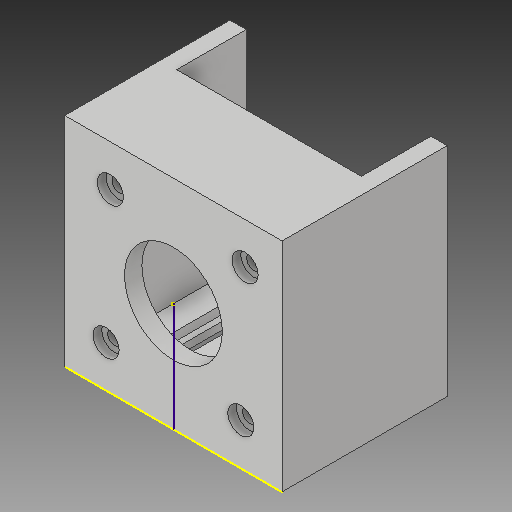
# Autodesk Inventor part: stepperMount
Saved by Autodesk Inventor 2017 (Build 210142000, 142)
## iProperties
Created: 2017-04-11
Part Number: stepperMount
Material: Generic
Document SubType Name: Modeling
Designer: Andres Celi
Density: 1 g/cm^3
Appearance: Default
Author: Andres Celi
Autodesk Inventor part; units mm, degrees
ref_plane "YZ Plane" through (0, 0, 0) normal (1, 0, 0) x (0, 1, 0)
ref_plane "XZ Plane" through (0, 0, 0) normal (0, 1, 0) x (-1, 0, 0)
ref_plane "XY Plane" through (0, 0, 0) normal (0, 0, 1) x (1, 0, 0)
sketch "Sketch1" plane through (0, 0, 0) normal (0, 0, 1) x (1, 0, 0)
  point P0 (0, 0)
sketch "Sketch2" plane through (0, 0, 0) normal (0, 0, 1) x (1, 0, 0)
  line L0 (-25, 25) -> (25, 25)
  line L1 (25, 25) -> (25, -25)
  line L2 (25, -25) -> (-25, -25)
  line L3 (-25, -25) -> (-25, 25)
  point P0 (0, 0)
  dimension "d0" = 50
  dimension "d1" = 50
  dimension "d2" = 25
  dimension "d3" = 25
  constraints: 8 end point, 2 parallel, 1 horizontal, 1 perpendicular
  measures "d0" distance of L1.end L2.end
  measures "d1" distance of L0.end L1.end
  measures "d2" distance from line of L3 point (0, 0)
  measures "d3" distance from line of point (0, 0) L0
extrude "Extrusion1" add sketch "Sketch2" along normal blind 38
sketch "Sketch3" plane through (0, 0, 0) normal (0, 0, -1) x (-1, 0, 0)
  point P0 (0, 0)
sketch "Sketch4" plane through (-25, 25, 0) normal (0, 1, 0) x (1, 0, 0)
  line L0 (0, 0) -> (50, 0) projected
  line L1 (46.25, 0) -> (3.75, 0)
  line L2 (3.75, 0) -> (3.75, -16)
  line L3 (3.75, -16) -> (46.25, -16)
  line L4 (46.25, -16) -> (46.25, 0)
  line L5 (50, 0) -> (50, -38) projected
  point P0 (25, 0)
  dimension "d6" = 42.5
  dimension "d7" = 16
  dimension "d8" = 3.75
  constraints: 8 end point, 2 parallel, 1 horizontal, 1 perpendicular, 1 point on line
  measures "d6" distance of L3.end L2.end
  measures "d7" distance of L2.end L1.end
  measures "d8" distance between parallel lines of L5 L4
extrude "Extrusion2" cut sketch "Sketch4" against normal blind 46.25
sketch "Sketch5" plane through (21.25, 25, 16) normal (0, 0, -1) x (-1, 0, 0)
  line L0 (0, -46.25) -> (0, 0) projected
  line L1 (42.5, 0) -> (42.5, -46.25) projected
  line L2 (0, -3.75) -> (42.5, -3.75)
  line L3 (42.5, -3.75) -> (42.5, -46.25)
  line L4 (42.5, -46.25) -> (0, -46.25)
  line L5 (0, -46.25) -> (0, -3.75)
  line L6 (-3.75, 0) -> (46.25, 0) projected
  point P0 (21.25, -25)
  dimension "d11" = 3.75
  constraints: 8 end point, 2 parallel, 1 horizontal, 1 perpendicular, 1 point on line
  measures "d11" distance between parallel lines of L6 L2
extrude "Extrusion3" cut sketch "Sketch5" against normal blind 18 contours L0 L2 L1 L4
sketch "Sketch6" plane through (-25, -25, 0) normal (-1, 0, 0) x (0, 0, 1)
  point P0 (0, 25)
sketch "Sketch7" plane through (0, 0, 38) normal (0, 0, 1) x (1, 0, 0)
  circle A0 centre (0, 0) radius 11.25
  dimension "d14" = 22.5
  constraints: 1 centre point, 1 coincident
  measures "d14" diameter of A0
extrude "Extrusion4" cut sketch "Sketch7" against normal blind 6
sketch "Sketch8" plane through (0, 0, 38) normal (0, 0, 1) x (1, 0, 0)
  circle A0 centre (-14.5105, 15.5) radius 1.625
  circle A1 centre (16.4895, 15.5) radius 1.625
  circle A2 centre (15.5, -15.5) radius 1.625
  circle A3 centre (-15.5, -15.5) radius 1.625
  point P0 (0, 0)
  dimension "d17" = 3.25
  dimension "d18" = 3.25
  dimension "d19" = 3.25
  dimension "d20" = 3.25
  dimension "d21" = 15.5
  dimension "d22" = 31
  dimension "d23" = 31
  dimension "d24" = 15.5
  dimension "d25" = 31
  dimension "d26" = 15.5
  dimension "d27" = 15.5
  constraints: 4 centre point
  measures "d17" diameter of A0
  measures "d18" diameter of A1
  measures "d19" diameter of A2
  measures "d20" diameter of A3
  measures "d21" vertical distance of point (0, 0) A0.centre
  measures "d22" vertical distance of A2.centre A1.centre
  measures "d23" distance of A0.centre A1.centre
  measures "d24" vertical distance of point (0, 0) A1.centre
  measures "d25" distance of A3.centre A2.centre
  measures "d26" horizontal distance of point (0, 0) A3.centre
  measures "d27" horizontal distance of point (0, 0) A3.centre
extrude "Extrusion5" cut sketch "Sketch8" against normal blind 4
sketch "Sketch9" plane through (-25, -21.25, 0) normal (0, 1, 0) x (1, 0, 0)
  point P0 (25, 0)
sketch "Sketch10" plane through (-25, -25, 0) normal (0, -1, 0) x (1, 0, 0)
  line L0 (37.5, 6.9021) -> (37.5, 27.0979) construction
  line L1 (46.25, 34) -> (3.75, 34) projected
  line L2 (39.125, 6.9021) -> (39.125, 27.0979)
  line L3 (35.875, 27.0979) -> (35.875, 6.9021)
  arc A0 (35.875, 6.9021) -> (39.125, 6.9021) centre (37.5, 6.9021) ccw
  arc A1 (39.125, 27.0979) -> (35.875, 27.0979) centre (37.5, 27.0979) ccw
  line L4 (12.5, 6.9021) -> (12.5, 27.0979) construction
  line L5 (14.125, 6.9021) -> (14.125, 27.0979)
  line L6 (10.875, 27.0979) -> (10.875, 6.9021)
  arc A2 (10.875, 6.9021) -> (14.125, 6.9021) centre (12.5, 6.9021) ccw
  arc A3 (14.125, 27.0979) -> (10.875, 27.0979) centre (12.5, 27.0979) ccw
  line L7 (50, 0) -> (0, 0) projected
  line L8 (0, 0) -> (0, 38) projected
  point P0 (25, 0)
  point P1 (37.5, 17)
  point P2 (12.5, 17)
  dimension "d30" = 3.25
  dimension "d31" = 3.25
  dimension "d32" = 17
  dimension "d33" = 17
  dimension "d34" = 25
  dimension "d35" = 12.5
  constraints: 16 end point, 8 point on circle, 8 tangent, 4 centre point, 3 parallel, 2 midpoint, 1 perpendicular
  measures "d30" diameter of A1
  measures "d31" diameter of A3
  measures "d32" distance from line of L7 point (37.5, 17)
  measures "d33" distance from line of L7 point (12.5, 17)
  measures "d34" distance of point (12.5, 17) point (37.5, 17)
  measures "d35" distance from line of L8 point (12.5, 17)
extrude "Extrusion6" cut sketch "Sketch10" against normal blind 4
sketch "Sketch11" plane through (0, 0, 38) normal (0, 0, 1) x (1, 0, 0)
  point P0 (0, 0)
sketch "Sketch12" plane through (0, 0, 38) normal (0, 0, 1) x (1, 0, 0)
  circle A0 centre (-14.5105, 15.5) radius 1.625 projected
  circle A1 centre (-14.5105, 15.5) radius 3
  circle A2 centre (16.4895, 15.5) radius 1.625 projected
  circle A3 centre (16.4895, 15.5) radius 3
  circle A4 centre (-15.5, -15.5) radius 1.625 projected
  circle A5 centre (-15.5, -15.5) radius 3
  circle A6 centre (15.5, -15.5) radius 1.625 projected
  circle A7 centre (15.5, -15.5) radius 3
  point P0 (0, 0)
  dimension "d38" = 6
  dimension "d39" = 6
  dimension "d40" = 6
  dimension "d41" = 6
  constraints: 4 centre point, 4 coincident
  measures "d38" diameter of A1
  measures "d39" diameter of A3
  measures "d40" diameter of A5
  measures "d41" diameter of A7
extrude "Extrusion7" cut sketch "Sketch12" against normal blind 2
sketch "Sketch13" plane through (-25, -21.25, 0) normal (0, 1, 0) x (1, 0, 0)
  arc A0 (10.875, -27.0979) -> (14.125, -27.0979) centre (12.5, -27.0979) ccw projected
  arc A1 (14.125, -6.9021) -> (10.875, -6.9021) centre (12.5, -6.9021) ccw projected
  line L0 (12.5, -27.0979) -> (12.5, -6.9021) construction
  line L1 (15.5, -27.0979) -> (15.5, -6.9021)
  line L2 (9.5, -6.9021) -> (9.5, -27.0979)
  arc A2 (9.5, -27.0979) -> (15.5, -27.0979) centre (12.5, -27.0979) ccw
  arc A3 (15.5, -6.9021) -> (9.5, -6.9021) centre (12.5, -6.9021) ccw
  arc A4 (35.875, -27.0979) -> (39.125, -27.0979) centre (37.5, -27.0979) ccw projected
  arc A5 (39.125, -6.9021) -> (35.875, -6.9021) centre (37.5, -6.9021) ccw projected
  line L3 (37.5, -27.0979) -> (37.5, -6.9021) construction
  line L4 (40.5, -27.0979) -> (40.5, -6.9021)
  line L5 (34.5, -6.9021) -> (34.5, -27.0979)
  arc A6 (34.5, -27.0979) -> (40.5, -27.0979) centre (37.5, -27.0979) ccw
  arc A7 (40.5, -6.9021) -> (34.5, -6.9021) centre (37.5, -6.9021) ccw
  point P0 (25, 0)
  point P1 (12.5, -17)
  point P2 (37.5, -17)
  dimension "d44" = 6
  dimension "d45" = 6
  constraints: 16 end point, 8 point on circle, 8 tangent, 4 centre point, 3 parallel, 2 midpoint, 1 vertical
  measures "d44" diameter of A3
  measures "d45" diameter of A7
extrude "Extrusion8" cut sketch "Sketch13" against normal blind 2
sketch "Sketch14" plane through (0, 0, 38) normal (0, 0, 1) x (1, 0, 0)
  line L0 (0, 0) -> (0, -25)
  line L1 (25, -25) -> (-25, -25) projected
  constraints: 2 end point, 1 midpoint
body "Solid1"
